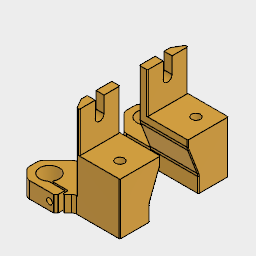
Z_Axis_Linear_Rail_Bracket_-_Double_Z_F01 (Autodesk Fusion 360 design; units mm, degrees)
Autodesk Fusion 360 part; units mm, degrees
sketch "スケッチ1" plane through (0, 0, 0) normal (0, 0, 1) x (1, 0, 0)
  circle A0 centre (0, 0) radius 6
  line L0 (19, 10) -> (-10, 10)
  line L1 (-10, 10) -> (-10, -15)
  line L2 (-10, -15) -> (47, -15)
  line L3 (47, -15) -> (47, 3.5)
  line L4 (47, 3.5) -> (19, 3.5)
  line L5 (19, 3.5) -> (19, 10)
  line L6 (15, 10) -> (15, 3.5)
  line L7 (14, 10) -> (14, 4.5)
  line L8 (19, 3.5) -> (12.5, 10)
  line L9 (19, 3.5) -> (28.1924, 3.5) construction
  line L10 (14, 4.5) -> (3.9686, 4.5)
  line L11 (15, 3.5) -> (4.8734, 3.5)
  circle A1 centre (37, -6.5) radius 5.25
  dimension "d1" = 12
  dimension "d2" = 10
  dimension "d3" = 10
  dimension "d4" = 15
  dimension "d5" = 47
  dimension "d6" = 3.5
  dimension "d7" = 28
  dimension "d8" = 1
  dimension "d9" = 25
  dimension "d10" = 135
  dimension "d11" = 1
  dimension "d12" = 6.5
  dimension "d13" = 10.5
  dimension "d15" = 10
  dimension "d66" = 10
  measures "d1" diameter of A0
  measures "d2" distance of A0.centre L0
  measures "d3" distance of A0.centre L1
  measures "d4" distance of A0.centre L2
  measures "d5" distance of A0.centre L3
  measures "d6" distance of A0.centre L4
  measures "d7" distance of L3 L5
  measures "d8" distance of L6 L7
  measures "d9" distance of L1 L6
  measures "d10" angle of L8 L9
  measures "d11" distance of L10 L11
  measures "d12" distance of L0 L11
  measures "d13" diameter of A1
  measures "d15" distance of L3 A1.centre
  measures "d66" distance of L4 A1.centre
extrude "押し出し1" add sketch "スケッチ1" along normal blind 10 contours A0 L0 L1 L2 L3 L4 L6 L7 L8 L10 L11 | A1 makes body 1
sketch "スケッチ2" plane through (47, 0, 0) normal (1, 0, 0) x (0, 1, 0)
  line L0 (-15, 0) -> (3.5, 0)
  line L1 (3.5, 0) -> (3.5, 10)
  line L2 (3.5, 10) -> (-15, 10)
  line L3 (-15, 10) -> (-15, 0)
  line L4 (3.5, 0) -> (3.5, 32)
  line L5 (3.5, 32) -> (-21.5, 32)
  line L6 (-21.5, 32) -> (-21.5, 27)
  line L7 (-21.5, 27) -> (-15, 10)
  line L8 (-15, 0) -> (3.5, 0)
  dimension "d18" = 32
  dimension "d19" = 25
  dimension "d20" = 5
  measures "d18" distance of L5 L8
  measures "d19" distance of L4 L6
  measures "d20" distance of L5.end L6.end
extrude "押し出し2" add sketch "スケッチ2" against normal blind 30 separate body makes body 2
sketch "スケッチ3" plane through (0, 0, 32) normal (0, 0, 1) x (-1, 0, 0)
  line L0 (-47, 21.5) -> (-47, -3.5)
  line L1 (-47, -3.5) -> (-17, -3.5)
  line L2 (-17, -3.5) -> (-17, 21.5)
  line L3 (-17, 21.5) -> (-47, 21.5)
  line L4 (-17, -3.5) -> (-22, -3.5)
  line L5 (-22, -3.5) -> (-22, 21.5)
  line L6 (-22, 21.5) -> (-17, 21.5)
  line L7 (-17, 21.5) -> (-17, -3.5)
  dimension "d23" = 5
  measures "d23" distance of L5 L7
extrude "押し出し3" add sketch "スケッチ3" along normal blind 25 contours L1 L2 L3 L4 L5 L6 L7 bodies 2
sketch "スケッチ4" plane through (0, 0, 32) normal (0, 0, 1) x (-1, 0, 0)
  line L0 (-22, -3.5) -> (-22, 21.5)
  line L1 (-22, 21.5) -> (-47, 21.5)
  line L2 (-47, 21.5) -> (-47, -3.5)
  line L3 (-47, -3.5) -> (-22, -3.5)
  circle A0 centre (-37, 6.5) radius 2.7
  dimension "d26" = 5.4
  dimension "d27" = 10
  dimension "d28" = 10
  measures "d26" diameter of A0
  measures "d27" distance of L3 A0.centre
  measures "d28" distance of L2 A0.centre
extrude "押し出し4" cut sketch "スケッチ4" against normal blind 4.6 contours A0 bodies 2
sketch "スケッチ6" plane through (22, 0, 0) normal (1, 0, 0) x (0, 1, 0)
  line L0 (-21.5, 32) -> (3.5, 32)
  line L1 (3.5, 32) -> (3.5, 57)
  line L2 (3.5, 57) -> (-21.5, 57)
  line L3 (-21.5, 57) -> (-21.5, 32)
  circle A0 centre (-9, 47) radius 2.7
  line L4 (3.5, 32) -> (-21.5, 32)
  line L5 (-11.7, 57) -> (-11.7, 47)
  line L6 (-6.3, 57) -> (-6.3, 47)
  dimension "d67" = 5.4
  dimension "d68" = 12.5
  dimension "d69" = 15
  measures "d67" diameter of A0
  measures "d68" distance of L3 A0.centre
  measures "d69" distance of A0.centre L4
extrude "押し出し9" cut sketch "スケッチ6" against normal blind 10 contours L2 A0 L5 L6 | A0 bodies 2
hole "穴2" at (10, 10, 5) direction (0, -1, 0) diameter 3.5 depth 30 tip angle 118 bodies 1
chamfer "面取り1" distance 3.5 distance2 6 1 edges at (17, 3.5, 28.5) measured on face at (28.6667, 3.5, 10.6667) on bodies 2
fillet "フィレット2" radius 5 2 edges at (32, -21.5, 27) (32, -15, 10) on bodies 2
fillet "フィレット3" radius 0.5 9 edges at (20.5, 3.5, 28.5) (17, -2.5, 28.5) (17, -15, 4.5384) (17, -15.0831, 9.9847) (17, -18.25, 18.5) (17, -21.4169, 27.0153) (17, -21.5, 42.4616) (22, -21.5, 44.5) (22, 3.5, 44.5) on bodies 2
fillet "フィレット4" radius 0.5 5 edges at (15, 7.5, 5) (14, 8.5, 5) (12.5, 10, 5) (4.8734, 3.5, 5) (3.9686, 4.5, 5) on bodies 1
fillet "フィレット5" radius 3 1 edges at (19, 3.5, 5) on bodies 1
chamfer "面取り2" distance 11 angle 45 1 edges at (-10, -15, 5) on bodies 1
chamfer "面取り3" distance 6 angle 45 1 edges at (-10, 10, 5) on bodies 1
fillet "フィレット6" radius 4 4 edges at (-4, 10, 5) (-10, 4, 5) (-10, -4, 5) (1, -15, 5) on bodies 1
sketch "スケッチ5" plane through (0, -15, 0) normal (0, -1, 0) x (1, 0, 0)
  circle A0 centre (10, 5) radius 1.75
  line L0 (2.6569, 10) -> (2.6569, 0)
  line L1 (2.6569, 0) -> (47, 0)
  line L2 (47, 0) -> (47, 10)
  line L3 (47, 10) -> (2.6569, 10)
  circle A1 centre (10, 5) radius 2.5
  circle A2 centre (10, 5) radius 2.35
  dimension "d55" = 5
  dimension "d56" = 4.7
  measures "d55" diameter of A1
  measures "d56" diameter of A2
extrude "押し出し6" cut sketch "スケッチ5" against normal blind 5 contours A2 bodies 1
extrude "押し出し7" cut sketch "スケッチ5" against normal blind 0.5 contours A1 bodies 1
combine "結合1" operation add target body 1 tool bodies 2
fillet "フィレット7" radius 0.5 6 edges at (47, -21.5, 29.9616) (47, -21.4169, 27.0153) (47, -18.25, 18.5) (47, -15.0831, 9.9847) (47, -15, 4.5384) (47, 3.5, 16) on bodies 1
extrude "押し出し8" cut sketch "スケッチ1" along normal blind 27 contours A1 bodies 1
ref_plane "作業平面1" through (0, -30, 0) normal (0, 1, 0) x (0, 0, 1)
mirror "ミラー1" about plane through (0, -30, 0) normal (0, 1, 0) of bodies 1 makes body 3
